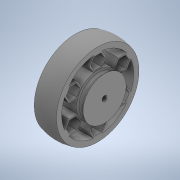
# Autodesk Inventor part: PulleyedWheelV1
Saved by Autodesk Inventor 2020 (Build 240168000, 168)
## iProperties
Created: 2023-12-21
Part Number: PulleyedWheelV1
Material: H TPU
Document SubType Name: Modeling
Designer: smz3rm
Density: 0.941117 g/cm^3
Appearance: Generic(1)
Mass: 15.2236 g
Surface Area: 99.7257 cm^2
Volume: 16.1761 cm^3
d0: 3.000 mm
d1: 1.000 mm
d3: 48.000 mm
d4: 3.000 mm
d6: 25.000 mm
d7: 4.000 mm
d8: 0.00 deg
d9: 48.000 mm
d10: 3.000 mm
d11: 0.800 mm
d12: 6.000 ul
d16: 13.000 mm
d17: 0.00 deg
d20: 2.000 mm
d24: 1.000 mm
d26: 45.00 deg
Roundedness: 1.000 mm
d14: 360.00 deg
BaseThickness: 3.000 mm
TopThickness: 1.000 mm
SideThickness: 6.000 mm
BodyWidth: 160.000 mm
BodyLength: 150.000 mm
BodyHeight: 35.000 mm
DriveMotorHeight: 17.500 mm
WheelDia: 50.000 mm
WheelWidth: 13.000 mm
WheelGrooveWidth: 4.000 mm
WheelGrooveDia: 25.000 mm
WheelSlotWidth: 20.000 mm
WheelPulleyDia: 2.000 mm
Author: smz3rm
Autodesk Inventor part; units mm, degrees
ref_plane "YZ Plane" through (0, 0, 0) normal (1, 0, 0) x (0, 1, 0)
ref_plane "XZ Plane" through (0, 0, 0) normal (0, 1, 0) x (-1, 0, 0)
ref_plane "XY Plane" through (0, 0, 0) normal (0, 0, 1) x (1, 0, 0)
sketch "Sketch1" plane through (0, 0, 0) normal (1, 0, 0) x (0, 1, 0)
  circle A0 centre (0, 0) radius 1.5
  line L0 (-33.6, 0) -> (33.6, 0) projected
  line L1 (1.118, -1) -> (-1.118, -1)
  circle A1 centre (0, 0) radius 12.5
  circle A2 centre (0, 0) radius 24
  circle A3 centre (0, 0) radius 21
  dimension "d0" = 3
  dimension "d1" = 1
  dimension "d3" = 48
  dimension "d4" = 3
  dimension "d6" = 25
  constraints: 4 centre point, 4 coincident, 2 end point, 2 point on circle, 1 horizontal
  measures "d0" diameter of A0
  measures "d1" distance between parallel lines of L0 L1
  measures "d3" diameter of A2
  measures "d4" radial gap between concentric circles of A2 A3
  measures "d6" diameter of A1
extrude "Extrusion1" add sketch "Sketch1" along normal blind 4 contours L1 A0 | A0 L0 A1 | L0 A1 A0
sketch "Sketch3" plane through (0, 0, 0) normal (0, 0, 1) x (1, 0, 0)
  line L0 (0, 12.5) -> (4, 12.5) projected
  line L1 (-0.8, 0) -> (4.8, 0) projected
  circle A0 centre (1.3858, 11.5) radius 1
  line L2 (0.4001, 11.3312) -> (0.2, 12.5)
  line L3 (0, 12.5) -> (4, 12.5) projected
  line L4 (0, 10) -> (4, 10) projected
  line L5 (0, 12.5) -> (4, 12.5) projected
  line L6 (3.8, 12.5) -> (2.0929, 10.7929)
  line L7 (3.8, 12.5) -> (3.8, 12.5)
  line L8 (3.8, 12.5) -> (4, 12.5)
  line L9 (4, -12.5) -> (4, 12.5) projected
  line L10 (4, 12.5) -> (4, 12.5)
  line L11 (0, -12.5) -> (0, 12.5) projected
  line L12 (0.2, 12.5) -> (0, 12.5)
  point P0 (0, 0)
  point P1 (1.3858, 12.5)
  point P2 (3.8, 12.5)
  dimension "d20" = 2
  dimension "d26" = 45
  dimension "d28" = 0.2
  constraints: 12 end point, 3 perpendicular, 3 tangent, 2 collinear, 2 point on circle, 2 point on line, 1 centre point, 1 vertical, 3 other
  measures "d20" diameter of A0
  measures "d26" angle of L0 L6
  measures "d28" distance of L0.end L6.start
revolve "Revolution1" cut sketch "Sketch3" angle 360 about axis through (-10, 0, 0) along (-1, 0, 0) contours L0 A0 L2 | L0 L6 A0 | A0
sketch "Sketch2" plane through (0, 0, 0) normal (-1, 0, 0) x (0, 0, 1)
  circle A0 centre (0, 0) radius 24
  circle A1 centre (0, 0) radius 21
  circle A2 centre (0, 0) radius 12.5 projected
  line L0 (-1, 1.118) -> (-1, -1.118) projected
  arc A3 (-1, -1.118) -> (-1, 1.118) centre (0, 0) ccw projected
  line L1 (2.4831, 20.8527) -> (4.9662, 16.5518)
  line L2 (4.9662, 16.5518) -> (2.4831, 12.2509)
  line L3 (2.4831, 12.2509) -> (-2.4831, 12.2509)
  line L4 (-2.4831, 12.2509) -> (-4.9662, 16.5518)
  line L5 (-4.9662, 16.5518) -> (-2.4831, 20.8527)
  line L6 (-2.4831, 20.8527) -> (2.4831, 20.8527)
  line L7 (0, -33.6) -> (0, 33.6) projected
  line L8 (-2.0212, 20.0527) -> (-4.0425, 16.5518)
  line L9 (-4.0425, 16.5518) -> (-2.0212, 13.0509)
  line L10 (-2.0212, 13.0509) -> (2.0212, 13.0509)
  line L11 (2.0212, 13.0509) -> (4.0425, 16.5518)
  line L12 (4.0425, 16.5518) -> (2.0212, 20.0527)
  line L13 (2.0212, 20.0527) -> (-2.0212, 20.0527)
  line L14 (-16.8174, 3.975) -> (-19.3005, 8.2759)
  line L15 (-11.8511, 3.975) -> (-16.8174, 3.975)
  line L16 (-9.368, 8.2759) -> (-11.8511, 3.975)
  line L17 (-19.3005, 8.2759) -> (-16.8174, 12.5768)
  line L18 (-16.8174, 12.5768) -> (-11.8511, 12.5768)
  line L19 (-11.8511, 12.5768) -> (-9.368, 8.2759)
  line L20 (-16.3555, 11.7768) -> (-18.3767, 8.2759)
  line L21 (-18.3767, 8.2759) -> (-16.3555, 4.775)
  line L22 (-16.3555, 4.775) -> (-12.313, 4.775)
  line L23 (-12.313, 4.775) -> (-10.2918, 8.2759)
  line L24 (-10.2918, 8.2759) -> (-12.313, 11.7768)
  line L25 (-12.313, 11.7768) -> (-16.3555, 11.7768)
  line L26 (-11.8511, -12.5768) -> (-16.8174, -12.5768)
  line L27 (-9.368, -8.2759) -> (-11.8511, -12.5768)
  line L28 (-11.8511, -3.975) -> (-9.368, -8.2759)
  line L29 (-16.8174, -12.5768) -> (-19.3005, -8.2759)
  line L30 (-19.3005, -8.2759) -> (-16.8174, -3.975)
  line L31 (-16.8174, -3.975) -> (-11.8511, -3.975)
  line L32 (-18.3767, -8.2759) -> (-16.3555, -11.7768)
  line L33 (-16.3555, -11.7768) -> (-12.313, -11.7768)
  line L34 (-12.313, -11.7768) -> (-10.2918, -8.2759)
  line L35 (-10.2918, -8.2759) -> (-12.313, -4.775)
  line L36 (-12.313, -4.775) -> (-16.3555, -4.775)
  line L37 (-16.3555, -4.775) -> (-18.3767, -8.2759)
  line L38 (4.9662, -16.5518) -> (2.4831, -20.8527)
  line L39 (2.4831, -12.2509) -> (4.9662, -16.5518)
  line L40 (-2.4831, -12.2509) -> (2.4831, -12.2509)
  line L41 (2.4831, -20.8527) -> (-2.4831, -20.8527)
  line L42 (-2.4831, -20.8527) -> (-4.9662, -16.5518)
  line L43 (-4.9662, -16.5518) -> (-2.4831, -12.2509)
  line L44 (-2.0212, -20.0527) -> (2.0212, -20.0527)
  line L45 (2.0212, -20.0527) -> (4.0425, -16.5518)
  line L46 (4.0425, -16.5518) -> (2.0212, -13.0509)
  line L47 (2.0212, -13.0509) -> (-2.0212, -13.0509)
  line L48 (-2.0212, -13.0509) -> (-4.0425, -16.5518)
  line L49 (-4.0425, -16.5518) -> (-2.0212, -20.0527)
  line L50 (16.8174, -3.975) -> (19.3005, -8.2759)
  line L51 (11.8511, -3.975) -> (16.8174, -3.975)
  line L52 (9.368, -8.2759) -> (11.8511, -3.975)
  line L53 (19.3005, -8.2759) -> (16.8174, -12.5768)
  line L54 (16.8174, -12.5768) -> (11.8511, -12.5768)
  line L55 (11.8511, -12.5768) -> (9.368, -8.2759)
  line L56 (16.3555, -11.7768) -> (18.3767, -8.2759)
  line L57 (18.3767, -8.2759) -> (16.3555, -4.775)
  line L58 (16.3555, -4.775) -> (12.313, -4.775)
  line L59 (12.313, -4.775) -> (10.2918, -8.2759)
  line L60 (10.2918, -8.2759) -> (12.313, -11.7768)
  line L61 (12.313, -11.7768) -> (16.3555, -11.7768)
  line L62 (11.8511, 12.5768) -> (16.8174, 12.5768)
  line L63 (9.368, 8.2759) -> (11.8511, 12.5768)
  line L64 (11.8511, 3.975) -> (9.368, 8.2759)
  line L65 (16.8174, 12.5768) -> (19.3005, 8.2759)
  line L66 (19.3005, 8.2759) -> (16.8174, 3.975)
  line L67 (16.8174, 3.975) -> (11.8511, 3.975)
  line L68 (18.3767, 8.2759) -> (16.3555, 11.7768)
  line L69 (16.3555, 11.7768) -> (12.313, 11.7768)
  line L70 (12.313, 11.7768) -> (10.2918, 8.2759)
  line L71 (10.2918, 8.2759) -> (12.313, 4.775)
  line L72 (12.313, 4.775) -> (16.3555, 4.775)
  line L73 (16.3555, 4.775) -> (18.3767, 8.2759)
  point P0 (0, 16.5518)
  point P1 (-2.4831, -20.8527)
  point P2 (-9.368, -8.2759)
  point P3 (-2.4831, -12.2509)
  point P4 (-9.368, 8.2759)
  point P5 (-16.8174, 12.5768)
  point P6 (16.8174, 12.5768)
  point P7 (9.368, 8.2759)
  point P8 (2.4831, 12.2509)
  point P9 (19.3005, -8.2759)
  point P10 (11.8511, -3.975)
  point P11 (11.8511, 3.975)
  point P12 (19.3005, 8.2759)
  point P13 (2.4831, -20.8527)
  point P14 (2.4831, -12.2509)
  point P15 (9.368, -8.2759)
  point P16 (-19.3005, 8.2759)
  point P17 (-11.8511, -3.975)
  point P18 (-19.3005, -8.2759)
  dimension "d9" = 48
  dimension "d10" = 3
  dimension "d11" = 0.8
  dimension "d14" = 360
  constraints: 144 end point, 2 centre point, 2 coincident, 2 point on circle, 1 point on line, 165 other
  measures "d9" diameter of A0
  measures "d10" radial gap between concentric circles of A0 A1
  measures "d11" distance between parallel lines of L5 L8
extrude "Extrusion2" add sketch "Sketch2" along normal blind 13 contours A0 L7 A1 | L7 A1 A0 | L7 L6 A1 | A1 L6 L7 | L7 L41 A1 | A1 L41 L7 | L1 L2 A2 L7 L10 L11 L12 L13 L6 | L6 L7 L13 L8 L9 L10 A2 L4 L5 | L42 L43 A2 L7 L47 L48 L49 L44 L41 | L41 L7 L44 L45 L46 L47 A2 L39 L38 | L65 L66 L67 A2 L63 L62 | A1 L65 | L17 A1 | L18 L19 A2 L15 L14 L17 | L29 L30 L31 A2 L27 L26 | A1 L29 | L53 A1 | L54 L55 A2 L51 L50 L53 | L3 L7 A2 | A2 L64 L52 L40 L7 A3 L3 | L3 L7 A3 L0 L40 A2 L28 L16 | A2 L7 L3 | L40 L7 A2 | A2 L7 L40 | A2 L64 | L16 A2 | A2 L28 | L52 A2
sketch "Sketch4" plane through (0, 0, 0) normal (0, 0, 1) x (1, 0, 0)
  line L0 (0, 24) -> (-13, 24) projected
  line L1 (-13, 24) -> (-13, -24) projected
  arc A0 (0, 24) -> (-13, 24) centre (-6.5, 3.375) ccw
  line L2 (-15.6, 0) -> (2.6, 0) projected
  point P0 (0, 0)
  point P1 (-6.5, 25)
  dimension "d24" = 1
  constraints: 3 point on circle, 1 centre point
  measures "d24" distance from line of L0 point (-6.5, 25)
revolve "Revolution2" add sketch "Sketch4" angle 360 about axis through (-10, 0, 0) along (1, 0, 0)
equation "\"d6\" = WheelGrooveDia"
equation "\"d7\" = WheelGrooveWidth"
equation "\"d20\" = WheelPulleyDia"
equation "\"d9\" = WheelDia - 2 * Roundedness"
equation "\"d16\" = WheelWidth"
equation "\"d24\" = Roundedness"
equation "\"Roundedness\" = 1"
equation "\"WheelGrooveDia\" = 25"
equation "\"WheelGrooveWidth\" = 4"
equation "\"WheelPulleyDia\" = 2"
equation "\"WheelDia\" = 50"
equation "\"WheelWidth\" = 13"
body "Solid1"
